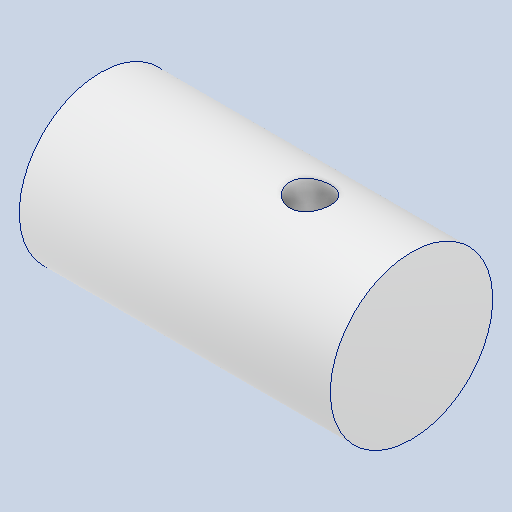
# Autodesk Inventor part: roller-hand-v2-Shaft-m-r
Saved by Autodesk Inventor 2025.1 (Build 291241000, 241)
## iProperties
Created: 2024-10-06
Part Number: roller-hand-v2-Shaft-m-r
Material: アルミニウム 6061
Document SubType Name: Modeling
Designer: haruy
Density: 2.7 g/cm^3
Appearance: アルミニウム - フラット
Author: haruy
Autodesk Inventor part; units mm, degrees
ref_plane "YZ Plane" through (0, 0, 0) normal (1, 0, 0) x (0, 1, 0)
ref_plane "XY Plane" through (0, 0, 0) normal (0, 0, 1) x (1, 0, 0)
sketch "スケッチ1" plane through (0, 0, 0) normal (1, 0, 0) x (0, 1, 0)
  circle A0 centre (0, 0) radius 6
  dimension "d0" = 12
  constraints: 1 centre point, 1 coincident
  measures "d0" diameter of A0
extrude "押し出し1" add sketch "スケッチ1" along normal blind 23
ref_plane "作業平面1" through (0, 6, 0) normal (0, 1, 0) x (-1, 0, 0)
sketch "スケッチ2" plane through (0, 6, 0) normal (0, 1, 0) x (-1, 0, 0)
  line L0 (0, 6) -> (0, -6) projected
  line L1 (-23, 6) -> (-23, -6) projected
  point P0 (0, 0)
  point P1 (-15.5, 0)
  dimension "d11" = 7.5
  measures "d11" distance from line of point (-15.5, 0) L1
hole "穴1" at (15.5, 6, 0) direction (0, -1, 0) diameter 3 end through all
